Autodesk Inventor part; units mm, degrees
(part 2 of 2)
  circle A64 centre (3635.4766, -1445.1584) radius 4.8387 projected
  circle A65 centre (3635.4766, -1445.1584) radius 4.8387 projected
  circle A66 centre (3654.8314, -1445.1584) radius 4.8387 projected
  circle A67 centre (3674.1862, -1445.1584) radius 4.8387 projected
  circle A68 centre (3674.1862, -1445.1584) radius 4.8387 projected
  circle A69 centre (3693.541, -1445.1584) radius 4.8387 projected
  circle A70 centre (3693.541, -1445.1584) radius 4.8387 projected
  circle A71 centre (3712.8958, -1445.1584) radius 4.8387 projected
  circle A72 centre (3712.8958, -1445.1584) radius 4.8387 projected
  circle A73 centre (3654.8314, -1445.1584) radius 4.8387 projected
  circle A74 centre (3848.3794, -1516.126) radius 4.8387 projected
  circle A75 centre (3848.3794, -1516.126) radius 4.8387 projected
  circle A76 centre (3848.3794, -1535.4808) radius 4.8387 projected
  circle A77 centre (3848.3794, -1535.4808) radius 4.8387 projected
  circle A78 centre (3848.3794, -1554.8356) radius 4.8387 projected
  circle A79 centre (3848.3794, -1554.8356) radius 4.8387 projected
  arc A80 (3852.944, -1575.7959) -> (3843.8148, -1575.7959) centre (3848.3794, -1574.1904) ccw projected
  circle A81 centre (3848.3794, -1496.7712) radius 4.8387 projected
  circle A82 centre (3848.3794, -1496.7712) radius 4.8387 projected
  circle A83 centre (3848.3794, -1470.9648) radius 4.8387 projected
  circle A84 centre (3848.3794, -1470.9648) radius 4.8387 projected
  circle A85 centre (3848.3794, -1445.1584) radius 4.8387 projected
  circle A86 centre (3848.3794, -1445.1584) radius 4.8387 projected
  circle A87 centre (3829.0246, -1445.1584) radius 4.8387 projected
  circle A88 centre (3829.0246, -1445.1584) radius 4.8387 projected
  circle A89 centre (3809.6698, -1445.1584) radius 4.8387 projected
  circle A90 centre (3790.315, -1445.1584) radius 4.8387 projected
  circle A91 centre (3790.315, -1445.1584) radius 4.8387 projected
  circle A92 centre (3770.9602, -1445.1584) radius 4.8387 projected
  circle A93 centre (3770.9602, -1445.1584) radius 4.8387 projected
  circle A94 centre (3751.6054, -1445.1584) radius 4.8387 projected
  circle A95 centre (3751.6054, -1445.1584) radius 4.8387 projected
  circle A96 centre (3732.2506, -1445.1584) radius 4.8387 projected
  circle A97 centre (3732.2506, -1445.1584) radius 4.8387 projected
  circle A98 centre (3809.6698, -1445.1584) radius 4.8387 projected
  circle A99 centre (3461.2834, -1445.1584) radius 4.8387 projected
  circle A100 centre (3461.2834, -1445.1584) radius 4.8387 projected
  circle A101 centre (3480.6382, -1445.1584) radius 4.8387 projected
  circle A102 centre (3480.6382, -1445.1584) radius 4.8387 projected
  circle A103 centre (3499.993, -1445.1584) radius 4.8387 projected
  circle A104 centre (3499.993, -1445.1584) radius 4.8387 projected
  circle A105 centre (3519.3478, -1445.1584) radius 4.8387 projected
  circle A106 centre (3538.7026, -1445.1584) radius 4.8387 projected
  circle A107 centre (3538.7026, -1445.1584) radius 4.8387 projected
  circle A108 centre (3558.0574, -1445.1584) radius 4.8387 projected
  circle A109 centre (3558.0574, -1445.1584) radius 4.8387 projected
  circle A110 centre (3577.4122, -1445.1584) radius 4.8387 projected
  circle A111 centre (3577.4122, -1445.1584) radius 4.8387 projected
  circle A112 centre (3519.3478, -1445.1584) radius 4.8387 projected
  point P0 (0, 0)
  point P1 (3538.4642, -1575.7959)
  constraints: 2 other
extrude "Extrusion1" add sketch "Sketch1" along normal blind 0.0025 contours L22 L23 L24 L25 L26 L27 L28 L29 L30 L31 L32 L33 L34 L35 L36 L37 L38 L39 L40 L41 L42 L43 L44 L45 L46 L47 L48 L49 L50 L51 L52 L53 L54 L55 L56 L57 L58 L59 L60 L61 L62 L63 L64 L65 L66 L67 L68 L69 L70 L71 L72 L73 L74 L75 L76 L77 L78 L79 L80 L81 L82 L83 L84 L85 L86 L87 L88 L89 L90 L91 L92 L93 L94 L95 L96 L97 L98 L99 L100 L101 L102 L103 L104 L105 L106 L107 L108 L109 L110 L111 L112 L113 L114 L115 L116 L117 L118 L119 L120 L121 L122 L123 L124 L125 L126 L127 L128 L129 L130 L131 L132 L133 L134 L135 L136 L137 L138 L139 L140 L141 L142 L143 L144 L145 L146 L147 L148 L149 L150 L151 L152 L153 L154 L155 L156 L157 L158 L159 L160 L161 L162 L163 L164 L165 L166 L167 L168 L169 L170 L171 L172 L173 L174 L175 L176 L177 L178 L179 L180 L181 L182 L183 L184 L185 L186 L187 L188 L189 L190 L191 L192 L193 L194 L195 L196 L197 L198 L199 L200 L201 L202 L203 L204 L205 L206 L207 L208 L209 L210 L211 L212 L213 L214 L215 L216 L217 L218 L219 L220 L221 L222 L223 L224 L225 L226 L227 L228 L229 L230 L231 L232 L233 L234 L235 L236 L237 L238 L670 L671 L672 L641 L642 L643 L644 L645 L646 L647 L648 L649 L650 L651 L652 L653 L654 L655 L656 L657 L658 L659 L660 L661 L662 L663 L664 L665 L666 L667 L668 L669 A80 | L670 L730 L729 L728 L727 L726 L725 L724 L723 L722 L721 L720 L719 L718 L717 L716 L715 L714 L713 L712 L711 L710 L709 L708 L707 L706 L705 L704 L703 L702 L701 L700 L699 L698 L697 L696 L695 L694 L693 L692 L691 L690 L689 L688 L687 L686 L685 L684 L683 L682 L681 L680 L679 L678 L677 L676 L675 L674 | L670 L588 L587 L586 L585 L584 L583 L582 L581 L580 L579 L578 L577 L576 L575 L574 L573 L572 L571 L570 L569 L568 L567 L566 L565 L564 L563 L562 L561 L560 L559 L558 L557 L556 L555 L554 L553 L552 L551 L550 L549 L548 L547 L546 L545 L544 L543 L542 L541 L540 L539 L538 L537 L536 L535 L534 L533 L532 L531 L530 L529 L528 L527 L526 L525 L524 L523 L522 L521 L520 L519 L518 L517 L516 L515 L514 L513 L512 L511 L510 L509 L508 L507 L506 L505 L504 L503 L502 L501 L500 L499 L498 L497 L496 L495 L494 L493 L492 L491 L490 L489 L488 L487 L486 L485 L484 L483 L482 L481 L480 L479 L478 L477 L476 L475 L474 L473 L472 L471 L470 L469 L468 L467 L466 L465 L464 L463 L462 L461 L460 L459 L458 L457 L456 L455 L454 L453 L452 L451 L450 L449 L448 L447 L446 L445 L444 L443 L442 L441 L440 L439 L438 L437 L436 L435 L434 L433 L431 L430 L429 L428 L427 L426 L425 L424 L423 L422 L421 L420 L419 L418 L417 L416 L415 L414 L413 L412 L411 L410 L409 L408 L407 L406 L405 L404 L403 L402 L401 L400 L399 L398 L397 L396 L395 L394 L393 L392 L391 L390 L389 L388 L387 L386 L385 L384 L383 L382 L381 L380 L379 L378 L377 L376 L375 L374 L373 L372 L371 L370 L369 L368 L367 L366 L365 L364 L363 L362 L361 L360 L359 L358 L357 L356 L355 L354 L353 L352 L351 L350 L349 L348 L347 L346 L345 L344 L343 L342 L341 L340 L339 L338 L337 L336 L335 L334 L333 L332 L331 L330 L329 L328 L327 L326 L325 L324 L323 L322 L321 L320 L319 L318 L317 L316 L315 L314 L313 L312 L311 L310 L309 L308 L307 L306 L305 L304 L303 L302 L301 L300 L299 L298 L297 L296 L295 L294 L293 L292 L291 | L670 L611 L612 L613 L614 L615 L616 L617 L618 L619 L620 L621 L622 L623 L624 L625 L626 L627 L628 L629 L630 L631 L632 L633 L634 L635 L636 L637 L638 L639 L640 | L239 L240 L241 L242 L243 L244 L245 L246 L247 L248 L249 L250 L251 L252 L253 L254 L255 L256 L257 L258 L259 L260 L261 L262 L263 L264 L265 L266 L267 L268 L269 L270 L271 L272 L273 L274 L275 L276 L277 L278 L279 L280 L281 L282 L283 L284 L285 L286 L287 L288 L289 L290
body "Solid1"
